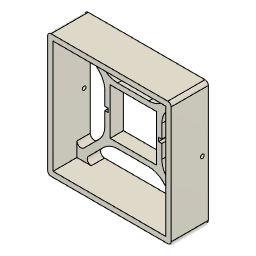
PCB Holder v9 (Autodesk Fusion 360 design; units mm, degrees)
Autodesk Fusion 360 part; units mm, degrees
note: some values were not read from the file. Set by a fixed rule: which sketch regions a step uses.
sketch "Sketch1" plane through (0, 0, 0) normal (0, 0, 1) x (1, 0, 0)
  line L0 (17.45, 17.45) -> (-17.45, 17.45)
  line L1 (-17.45, 17.45) -> (-17.45, -17.45)
  line L2 (-17.45, -17.45) -> (17.45, -17.45)
  line L3 (17.45, -17.45) -> (17.45, 17.45)
  line L4 (17.45, 17.45) -> (-17.45, -17.45) construction
  line L5 (-17.45, 17.45) -> (17.45, -17.45) construction
  line L6 (-21.45, -21.45) -> (21.45, -21.45)
  line L7 (21.45, -21.45) -> (21.45, 21.45)
  line L8 (21.45, 21.45) -> (-21.45, 21.45)
  line L9 (-21.45, 21.45) -> (-21.45, -21.45)
  line L10 (-42.45, -42.45) -> (42.45, -42.45)
  line L11 (42.45, -42.45) -> (42.45, 42.45)
  line L12 (42.45, 42.45) -> (-42.45, 42.45)
  line L13 (-42.45, 42.45) -> (-42.45, -42.45)
  line L14 (-46.45, 46.45) -> (-46.45, -46.45)
  line L15 (-46.45, -46.45) -> (46.45, -46.45)
  line L16 (46.45, -46.45) -> (46.45, 46.45)
  line L17 (46.45, 46.45) -> (-46.45, 46.45)
  line L18 (-42.45, -42.45) -> (-17.45, -17.45)
  line L19 (17.45, -17.45) -> (42.45, -42.45)
  line L20 (17.45, 17.45) -> (42.45, 42.45)
  line L21 (-17.45, 17.45) -> (-42.45, 42.45)
  line L22 (-15.6822, 19.2178) -> (-40.6822, 44.2178)
  line L23 (-19.2178, 15.6822) -> (-44.2178, 40.6822)
  line L24 (-40.6822, -44.2178) -> (-15.6822, -19.2178)
  line L25 (-44.2178, -40.6822) -> (-19.2178, -15.6822)
  line L26 (15.6822, -19.2178) -> (40.6822, -44.2178)
  line L27 (19.2178, -15.6822) -> (44.2178, -40.6822)
  line L28 (19.2178, 15.6822) -> (44.2178, 40.6822)
  line L29 (15.6822, 19.2178) -> (40.6822, 44.2178)
  dimension "d1" = 34.9
  dimension "d2" = 34.9
  dimension "d3" = 4
  dimension "d20" = 25
  dimension "d21" = 29
  dimension "d22" = 2.5
  dimension "d23" = -2.5
  dimension "d24" = 2.5
  dimension "d25" = -2.5
  dimension "d26" = 2.5
  dimension "d27" = -2.5
  dimension "d28" = 2.5
  dimension "d29" = -2.5
  constraint horizontal L0
  constraint perpendicular L0 L1
  constraint parallel L0 L2
  constraint parallel L1 L3
  constraint coincident L4 origin
  constraint coincident L5 origin
  measures "d1" distance of L1.end L2.end
  measures "d2" distance of L0.end L1.end
extrude "Extrude1" add sketch "Sketch1" along normal blind 10 contours L3 L7 L19 L20 | L0 L8 L20 L21 | L1 L9 L18 L21 | L2 L6 L18 L19
extrude "Extrude5" add sketch "Sketch1" along normal up to surface (10 mm away) contours L7 L11 L20 L28 | L8 L12 L20 L29 | L8 L12 L21 L22 | L9 L13 L21 L23 | L6 L10 L19 L26 | L7 L11 L19 L27 | L9 L13 L18 L25 | L6 L10 L18 L24 | L14 L15 L16 L17
extrude "Extrude6" add sketch "Sketch1" along normal blind 28
sketch "Sketch4" plane through (-46.45, 0, 0) normal (-1, 0, 0) x (0, 0, 1)
  line L0 (0, 46.45) -> (0, -46.45)
  line L1 (28, -46.45) -> (28, 46.45)
  circle A0 centre (4.5, 0) radius 1.4
  line L2 (28, 46.45) -> (0, 46.45)
  line L3 (0, -46.45) -> (28, -46.45)
  line L4 (4.5, 1.4) -> (10.2364, 1.4)
  line L5 (10.2364, 1.4) -> (10.2364, -1.4)
  line L6 (10.2364, -1.4) -> (4.5, -1.4)
  line L7 (4.5, -1.4) -> (4.5, 1.4)
  dimension "d42" = 2.8
  constraint horizontal L4
  constraint vertical L5
  constraint horizontal L6
  constraint vertical L7
  constraint coincident A0 L4.start
  constraint tangent A0 L6
  constraint tangent A0 L4
  constraint coincident L5.end L6.start
  measures "d42" diameter of A0
extrude "Extrude8" cut sketch "Sketch4" against normal up to surface (4 mm away) contours A0 L7 | A0 L7
extrude "Extrude13" cut sketch "Sketch4" against normal up to surface (4 mm away) from surface at -88.9 contours A0 L7 | A0 L7
extrude "Extrude15" cut sketch "Sketch4" against normal blind 2.5 from surface at -25 contours A0 L7 | A0 L4 L5 L6 | A0 L7
extrude "Extrude16" cut sketch "Sketch4" along normal blind 2.5 from surface at -67.9 contours A0 L7 | A0 L4 L5 L6 | A0 L7
fillet "Fillet7" radius 15 8 edges at (17.9145, 21.45, 5) (-17.9145, 21.45, 5) (-21.45, 17.9145, 5) (-21.45, -17.9145, 5) (-17.9145, -21.45, 5) (17.9145, -21.45, 5) (21.45, -17.9145, 5) (21.45, 17.9145, 5)
fillet "Fillet8" radius 3 8 edges at (38.9145, 42.45, 5) (42.45, 38.9145, 5) (42.45, -38.9145, 5) (38.9145, -42.45, 5) (-38.9145, -42.45, 5) (-42.45, -38.9145, 5) (-42.45, 38.9145, 5) (-38.9145, 42.45, 5)
fillet "Fillet9" radius 2.5 4 edges at (-46.45, -46.45, 14) (46.45, -46.45, 14) (46.45, 46.45, 14) (-46.45, 46.45, 14)
equation "d1 = d2"
equation "d20 = cageDistance"
equation "d21 = d20 + 4 mm"
equation "cageDistance = 25 mm"
